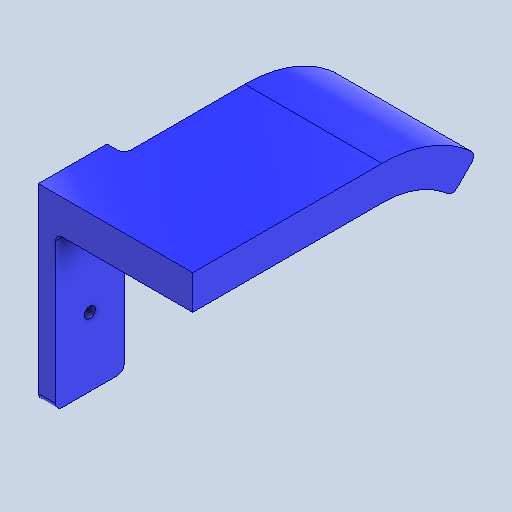
# Autodesk Inventor part: dribl-v4-3DP-2
Saved by Autodesk Inventor 2025.2 (Build 292293000, 293)
## iProperties
Created: 2025-05-17
Part Number: dribl-v4-3DP-2
Material: ABS プラスチック
Document SubType Name: Modeling
Designer: haruy
Density: 1.06 g/cm^3
Appearance: 青 - 壁塗料 - 光沢
Author: haruy
Autodesk Inventor part; units mm, degrees
ref_plane "YZ Plane" through (0, 0, 0) normal (1, 0, 0) x (0, 1, 0)
ref_plane "XZ Plane" through (0, 0, 0) normal (0, 1, 0) x (-1, 0, 0)
ref_plane "XY Plane" through (0, 0, 0) normal (0, 0, 1) x (1, 0, 0)
derived "dribl-v1-Plate-5.ipt"
sketch "スケッチ5" plane through (-210, -432.3334, -303) normal (-1, 0, 0) x (0, 0, 1)
  circle A0 centre (-55.18, 231) radius 16 projected
  line L0 (-20, 0) -> (-20, 1308) projected
  circle A1 centre (-55.18, 191) radius 16 projected
  line L1 (-20, 82) -> (-319.0594, 82) projected
  line L2 (-319.0594, 82) -> (-319.0594, 102) projected
  line L3 (-319.0594, 102) -> (-20, 102) projected
  line L4 (-20, 102) -> (-20, 82) projected
  line L5 (0, 0) -> (-20, 0) projected
  circle A2 centre (-55.18, 191) radius 9 projected
  line L6 (-55.18, 247) -> (0, 247) projected
  line L7 (-71.18, 231) -> (-71.18, 191) projected
  line L8 (-55.18, 175) -> (0, 175) projected
  line L9 (0, 1308) -> (0, 0) projected
  circle A3 centre (-10, 215) radius 1.5 construction
  circle A4 centre (-10, 195) radius 1.5 construction
  circle A5 centre (-55.18, 231) radius 6 projected
  line L10 (0, 230) -> (-20, 230)
  line L11 (0, 220) -> (-20, 220)
  circle A6 centre (-55.18, 191) radius 29
  line L12 (-20, 220) -> (-55.18, 220)
  line L13 (-55.18, 191) -> (-75.6861, 211.5061)
  line L14 (-55.18, 191) -> (-55.18, 220)
  circle A7 centre (-55.18, 191) radius 39
  line L15 (-20, 230) -> (-55.18, 230)
  line L16 (-55.18, 191) -> (-82.7572, 218.5772)
  circle A8 centre (-10, 215) radius 1.6
  circle A9 centre (-10, 195) radius 1.6
  point P0 (303, 432.3334)
  point P1 (-169.5297, 102)
  point P2 (-20, 175)
  point P3 (-75.6861, 211.5061)
  dimension "d1" = 15
  dimension "d2" = 10
  dimension "d3" = 45
  dimension "d4" = 10
  dimension "d5" = 3.2
  dimension "d6" = 3.2
  constraints: 14 end point, 6 point on line, 4 centre point, 4 point on circle, 3 coincident, 2 perpendicular, 1 horizontal, 1 tangent
  measures "d1" distance from line of A3.centre L10
  measures "d2" distance between parallel lines of L11 L10
  measures "d4" radial gap between concentric circles of A6 A7
  measures "d5" diameter of A8
  measures "d6" diameter of A9
extrude "押し出し1" add sketch "スケッチ5" along normal blind 5 contours L10 L9 L11 L0 | L11 L9 L8 A7 L0 | A7 L8 L0 picked at (-19.2978, 195.0889)
extrude "押し出し2" add sketch "スケッチ5" against normal blind 40 contours L15 L0 L12 A7 A0 | A0 A7 A5 L15 | A7 L12 A0 | A0 L12 A6 A7 A5 | L10 L9 L11 L0 | A5 A7 L15 | A0 A6 L7 A7 | L7 A6 L16 A7 | A5 A7 picked at (-44.8498, 229.6407) picked at (-51.2614, 229.9189)
fillet "フィレット1" radius 2 6 edges at (-212.5, -257.3334, -303) (-212.5, -257.3334, -323) (-210, -212.3334, -313) (-210, -207.3334, -323) (-190, -213.7562, -385.7572) (-190, -220.8273, -378.6861)
